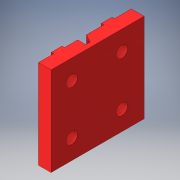
# Autodesk Inventor part: 80-20 extrusion rail
Saved by Autodesk Inventor 2016 SP2 (Build 200236200, 236)
## iProperties
Created: 2018-01-11
Part Number: 80-20 extrusion rail
Material: Generic
Document SubType Name: Modeling
Designer: CAD
Density: 1 g/cm^3
Appearance: Light Red
Author: CAD
Autodesk Inventor part; units mm, degrees
ref_plane "YZ Plane" through (0, 0, 0) normal (1, 0, 0) x (0, 1, 0)
ref_plane "XZ Plane" through (0, 0, 0) normal (0, 1, 0) x (-1, 0, 0)
ref_plane "XY Plane" through (0, 0, 0) normal (0, 0, 1) x (1, 0, 0)
sketch "Sketch1" plane through (0, 0, 0) normal (0, 1, 0) x (-1, 0, 0)
  line L0 (0, 0) -> (0, -52.6034)
  line L1 (0, -52.6034) -> (7.1438, -52.6034)
  line L2 (7.1438, -43.0784) -> (8.5408, -43.0784)
  line L3 (8.5408, -43.0784) -> (8.5408, -36.9824)
  line L4 (8.5408, -36.9824) -> (7.1437, -36.9824)
  line L5 (7.1438, -52.6034) -> (7.1438, -43.0784)
  line L6 (7.1437, -36.9824) -> (7.1437, -27.2034)
  line L7 (0, 0) -> (7.1437, 0)
  line L8 (7.1437, -22.225) -> (2.5207, -22.225)
  line L9 (2.5207, -22.225) -> (2.5207, -24.6063)
  line L10 (2.5207, -24.6063) -> (7.1437, -27.2034)
  line L11 (7.1437, -14.7574) -> (8.5407, -14.7574)
  line L12 (8.5407, -14.7574) -> (8.5407, -8.6614)
  line L13 (8.5407, -8.6614) -> (7.1437, -8.6614)
  line L14 (7.1437, 0) -> (7.1437, -8.6614)
  line L15 (7.1437, -14.7574) -> (7.1437, -22.225)
  dimension "d2" = 52.6034
  dimension "d3" = 7.1437
  dimension "d4" = 25.4
  dimension "d14" = 1.397
  dimension "d15" = 6.096
  dimension "d17" = 9.525
  dimension "d36" = 7.1437
  dimension "d41" = 22.225
  dimension "d42" = 2.3813
  dimension "d43" = 1.397
  dimension "d44" = 1.397
  dimension "d45" = 6.096
  dimension "d46" = 22.225
  dimension "d47" = 8.6614
  dimension "d48" = 4.6231
  constraints: 32 end point, 11 perpendicular, 3 horizontal, 2 vertical, 1 collinear
  measures "d2" distance of L0.start L0.end
  measures "d3" distance of L0.end L1.end
  measures "d4" distance of L1.end L6.end
  measures "d14" distance of L2.start L2.end
  measures "d15" distance of L2.end L3.end
  measures "d17" distance between parallel lines of L2 L1
  measures "d36" distance of L0.start L7.end
  measures "d41" distance of L7.end L8.start
  measures "d42" distance of L8.end L9.end
  measures "d43" distance of L11.start L11.end
  measures "d44" distance of L12.end L13.end
  measures "d45" distance of L11.end L12.end
  measures "d46" distance between parallel lines of L11 L4
  measures "d47" distance of L7.end L13.end
  measures "d48" horizontal distance of L9.end L6.end
extrude "Extrusion1" add sketch "Sketch1" along normal blind 50.292
sketch "Sketch3" plane through (-8.5408, 0, -43.0784) normal (-1, 0, 0) x (0, 0, 1)
  line L0 (6.096, 0) -> (6.096, 50.292) projected
  line L1 (0, 50.292) -> (6.096, 50.292) projected
  line L2 (0, 0) -> (6.096, 0) projected
  line L3 (34.417, 0) -> (34.417, 50.292) projected
  point P0 (43.0784, 0)
  point P1 (3.048, 39.1795)
  point P2 (3.048, 11.1125)
  point P3 (31.369, 39.1795)
  point P4 (31.369, 11.1125)
  dimension "d49" = 3.048
  dimension "d50" = 3.048
  dimension "d51" = 11.1125
  dimension "d52" = 11.1125
  dimension "d60" = 3.048
  dimension "d61" = 3.048
  dimension "d62" = 0
  dimension "d63" = 0
  measures "d49" distance from line of point (3.048, 39.18) L0
  measures "d50" distance from line of L0 point (3.048, 11.113)
  measures "d51" distance from line of L1 point (3.048, 39.18)
  measures "d52" distance from line of L2 point (3.048, 11.113)
  measures "d60" distance from line of L3 point (31.369, 11.113)
  measures "d61" distance from line of L3 point (31.369, 39.18)
  measures "d62" vertical distance of point (3.048, 39.18) point (31.369, 39.18)
  measures "d63" vertical distance of point (3.048, 11.113) point (31.369, 11.113)
hole "Hole2" at (-8.5408, 39.1795, -40.0304) at (-8.5408, 11.1125, -40.0304) at (-8.5408, 39.1795, -11.7094) at (-8.5408, 11.1125, -11.7094) direction (1, 0, 0) diameter 6.35 end through all
equation "\"d36\" = d3"
equation "\"d43\" = d14"
equation "\"d44\" = d14"
equation "\"d45\" = d15"
body "Solid1"
